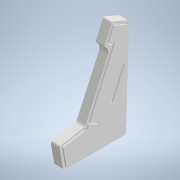
# Autodesk Inventor part: Arcade_Left
Saved by Autodesk Inventor 2022 (Build 260153000, 153)
## iProperties
Created: 2023-12-22
Part Number: Arcade_Left
Material: Generic
Document SubType Name: Modeling
Designer: Petr Černý
Density: 1 g/cm^3
Appearance: Default
Author: Petr Černý
Autodesk Inventor part; units mm, degrees
ref_plane "YZ Plane" through (0, 0, 0) normal (1, 0, 0) x (0, 1, 0)
ref_plane "XZ Plane" through (0, 0, 0) normal (0, 1, 0) x (-1, 0, 0)
ref_plane "XY Plane" through (0, 0, 0) normal (0, 0, 1) x (1, 0, 0)
sketch "Sketch1" plane through (0, 0, 0) normal (1, 0, 0) x (0, 1, 0)
  line L0 (0, 78.3368) -> (0, 427.0775)
  line L1 (9.8481, 428.814) -> (120.1519, 448.2635)
  line L2 (131.7365, 440.1519) -> (154.2135, 312.6787)
  line L3 (503.1119, 189.3047) -> (590.8645, 150.2346)
  line L4 (595.9326, 137.0318) -> (559.5861, 55.3964)
  line L5 (494.9423, 192.942) -> (494.9423, 192.942)
  line L6 (442.0149, 172.9748) -> (165.6696, 297.928)
  arc A0 (442.0149, 172.9748) -> (490.9347, 186.0198) centre (458.495, 209.4221) ccw
  arc A1 (154.2135, 312.6787) -> (165.6696, 297.928) centre (173.9096, 316.1516) ccw
  arc A2 (131.7365, 440.1519) -> (120.1519, 448.2635) centre (121.8884, 438.4154) ccw
  line L7 (9.8481, 428.814) -> (0, 417.0775)
  arc A3 (595.9326, 137.0318) -> (590.8645, 150.2346) centre (586.7972, 141.0991) ccw
  arc A4 (503.1119, 189.3047) -> (490.9347, 186.0198) centre (499.0446, 180.1692) ccw
  line L8 (9.651, 68.3429) -> (550.1017, 49.4699)
  arc A5 (550.1017, 49.4699) -> (559.5861, 55.3964) centre (550.4507, 59.4638) ccw
  arc A6 (0, 78.3368) -> (9.651, 68.3429) centre (10, 78.3368) ccw
  line L9 (0, 417.0775) -> (0, 78.3368)
  point P0 (534.922, 0)
  point P1 (130, 450)
  point P2 (156.0472, 302.2788)
  point P3 (600, 146.1672)
  point P4 (478.4622, 156.4947)
  point P5 (0, 427.0775)
  point P6 (0, 28.3368)
  dimension "d0" = 130
  dimension "d1" = 404.922
  dimension "d3" = 150
  dimension "d4" = 160
  dimension "d5" = 115
  dimension "d13" = 40
  dimension "d14" = 40
  dimension "d15" = 20
  dimension "d16" = 10
  dimension "d17" = 10
  dimension "d18" = 10
  dimension "d68" = 10
  dimension "d69" = 10
  constraints: 20 end point, 15 point on circle, 14 tangent, 13 point on line, 7 centre point, 3 perpendicular
  measures "d0" distance from line of point (130, 450) L0
  measures "d1" horizontal distance of point (130, 450) point (534.922, 0)
  measures "d3" distance of point (130, 450) point (156.047, 302.279)
  measures "d4" distance of point (600, 146.167) point (534.922, 0)
  measures "d5" distance of L5.start point (600, 146.167)
  measures "d13" distance of L5.start point (478.462, 156.495)
  measures "d14" radius of A0
  measures "d15" radius of A1
  measures "d16" radius of A2
  measures "d17" distance of L1.start point (0, 427.077)
  measures "d18" distance of L7.end point (0, 427.077)
  measures "d68" radius of A5
  measures "d69" radius of A6
extrude "Extrusion1" add sketch "Sketch1" along normal blind 16
sketch "Sketch2" plane through (16, 0, 0) normal (1, 0, 0) x (0, 0, -1)
  line L0 (-172.9748, 442.0149) -> (-297.928, 165.6696) projected
  line L1 (-428.814, 9.8481) -> (-417.0775, 0) projected
  line L2 (-417.0775, 0) -> (-78.3368, 0) projected
  line L3 (-55.3964, 559.5861) -> (-137.0318, 595.9326) projected
  arc A0 (-137.0318, 595.9326) -> (-150.2346, 590.8645) centre (-141.0991, 586.7972) ccw projected
  line L4 (-150.2346, 590.8645) -> (-189.3047, 503.1119) projected
  arc A1 (-189.3047, 503.1119) -> (-186.0198, 490.9347) centre (-180.1692, 499.0446) ccw projected
  arc A2 (-172.9748, 442.0149) -> (-186.0198, 490.9347) centre (-209.4221, 458.495) ccw projected
  line L5 (-172.9748, 442.0149) -> (-297.928, 165.6696) projected
  arc A3 (-312.6787, 154.2135) -> (-297.928, 165.6696) centre (-316.1516, 173.9096) ccw projected
  line L6 (-312.6787, 154.2135) -> (-440.1519, 131.7365) projected
  arc A4 (-440.1519, 131.7365) -> (-448.2635, 120.1519) centre (-438.4154, 121.8884) ccw projected
  line L7 (-448.2635, 120.1519) -> (-428.814, 9.8481) projected
  line L8 (-438.4154, 121.8884) -> (-310.9422, 144.3654)
  line L9 (-286.9073, 160.6932) -> (-163.5511, 437.7551)
  line L10 (-163.5511, 437.7551) -> (-143.4328, 482.9414)
  line L11 (-143.4328, 482.9414) -> (-139.4594, 491.8657)
  line L12 (-139.4594, 491.8657) -> (-130.324, 487.7983)
  line L13 (-130.324, 487.7983) -> (-288.9516, 131.5158)
  line L14 (-288.9516, 131.5158) -> (-298.087, 135.5831)
  line L15 (-298.087, 135.5831) -> (-286.9073, 160.6932)
  line L16 (-428.814, 9.8481) -> (-417.0775, 0) projected
  line L17 (-143.5969, 482.7615) -> (-143.5268, 482.7303)
  line L18 (-438.4154, 121.8884) -> (-303.4968, 145.6782)
  line L19 (-303.4968, 145.6782) -> (-301.7603, 135.8301)
  line L20 (-301.7603, 135.8301) -> (-436.679, 112.0403)
  line L21 (-438.4154, 121.8884) -> (-436.679, 112.0403)
  line L22 (-436.679, 112.0403) -> (-417.404, 2.7267)
  line L23 (-436.679, 112.0403) -> (-325.679, 112.0403) construction
  line L24 (-417.404, 2.7267) -> (-407.5559, 4.4631)
  line L25 (-407.5559, 4.4631) -> (-426.8309, 113.7768)
  line L26 (-141.0991, 586.7972) -> (-182.9931, 492.702)
  line L27 (-182.9931, 492.702) -> (-173.8576, 488.6347)
  line L28 (-173.8576, 488.6347) -> (-131.9637, 582.7298)
  line L29 (-139.4594, 491.8657) -> (-166.9664, 504.1126)
  line L30 (-139.4594, 491.8657) -> (-109.3492, 491.8657) construction
  line L31 (-166.9664, 504.1126) -> (-171.0338, 494.9772)
  line L32 (-171.0338, 494.9772) -> (-143.5268, 482.7303)
  line L33 (-141.0991, 586.7972) -> (-131.9637, 582.7298)
  line L34 (-131.9637, 582.7298) -> (3.0363, 582.7298) construction
  line L35 (-12.7024, 518.6849) -> (487.2976, 518.6849) construction
  line L36 (-288.9516, 131.5158) -> (-274.7158, 163.4898)
  line L37 (-274.7158, 163.4898) -> (-219.9031, 139.0856)
  line L38 (-219.9031, 139.0856) -> (-223.9704, 129.9501)
  line L39 (-223.9704, 129.9501) -> (-278.7831, 154.3544)
  line L40 (-68.3429, 9.651) -> (-49.4699, 550.1017) projected
  arc A5 (-49.4699, 550.1017) -> (-55.3964, 559.5861) centre (-59.4638, 550.4507) ccw projected
  arc A6 (-78.3368, 0) -> (-68.3429, 9.651) centre (-78.3368, 10) ccw projected
  line L41 (-131.9637, 582.7298) -> (-54.3123, 548.1572)
  line L42 (-131.9637, 582.7298) -> (-46.9637, 582.7298) construction
  line L43 (-54.3123, 548.1572) -> (-58.3797, 539.0217)
  line L44 (-136.0311, 573.5943) -> (-58.3797, 539.0217)
  line L45 (-170.9977, 396.4438) -> (-86.9516, 359.024)
  line L46 (-86.9516, 359.024) -> (-156.0969, 203.7213)
  line L47 (-156.0969, 203.7213) -> (-142.3938, 197.6203)
  line L48 (-142.3938, 197.6203) -> (-73.2484, 352.9229)
  line L49 (-73.2484, 352.9229) -> (-86.9516, 359.024)
  point P0 (0, 0)
  dimension "d25" = 10
  dimension "d26" = 390
  dimension "d27" = 10
  dimension "d37" = 137
  dimension "d38" = 111
  dimension "d39" = 80
  dimension "d40" = 10
  dimension "d41" = 90
  dimension "d42" = 90
  dimension "d43" = 103
  dimension "d44" = 10
  dimension "d45" = 90
  dimension "d46" = 156
  dimension "d60" = 35
  dimension "d61" = 60
  dimension "d62" = 90
  dimension "d63" = 10
  dimension "d64" = 90
  dimension "d65" = 90
  dimension "d70" = 85
  dimension "d71" = 24
  dimension "d72" = 92
  dimension "d73" = 100
  dimension "d74" = 170
  dimension "d75" = 15
  constraints: 80 end point, 12 point on line, 11 perpendicular, 5 horizontal, 3 equal length
  measures "d25" distance of L11.end L12.end
  measures "d26" distance of L12.end L13.end
  measures "d27" distance of L13.end L14.end
  measures "d37" distance of L8.start L18.end
  measures "d38" distance of L20.end L22.end
  measures "d39" angle of L22 L23
  measures "d40" distance of L22.end L24.end
  measures "d41" angle of L24 L22
  measures "d42" angle of L25 L24
  measures "d43" distance of L26.start L26.end
  measures "d44" distance of L26.end L27.end
  measures "d45" angle of L27 L26
  measures "d46" angle of L30 L29
  measures "d60" distance of L13.end L36.end
  measures "d61" distance of L36.end L37.end
  measures "d62" angle of L36 L37
  measures "d63" distance of L37.end L38.end
  measures "d64" angle of L37 L38
  measures "d65" angle of L38 L39
  measures "d70" distance of L33.end L41.end
  measures "d71" angle of L41 L42
  measures "d72" distance of L45.start L45.end
  measures "d73" distance between parallel lines of L12 L45
  measures "d74" distance of L45.end L46.end
  measures "d75" distance of L46.end L47.end
extrude "Extrusion2" cut sketch "Sketch2" against normal blind 7 contours L8 L18 L19 L20 L21 | L20 L25 L24 L22 | L9 L10 L11 L12 L13 L14 L15 | L17 L32 L28 L29 L11 L10 | L13 L37 L38 L39 | L28 L27 L26 L33 | L28 L41 L43 L44 | L49 L48 L47 L46
equation "\"d18\" = d17"
body "Solid1"
